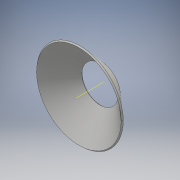
# Autodesk Inventor part: top_roof
Saved by Autodesk Inventor 2016 (Build 200138000, 138)
## iProperties
Created: 2018-04-03
Part Number: top_roof
Material: 一般
Document SubType Name: Sheet Metal
Designer: ASHIJANKEN
Density: 1 g/cm^3
Flat Pattern Width: 18.7953 cm
Flat Pattern Length: 18.7953 cm
Flat Pattern Area: 353.262 cm^2
Sheet Metal Rule: Default_mm
Sheet Metal Width: 187.953 mm
Sheet Metal Length: 187.953 mm
Sheet Metal Area: 35326.162 mm^2
Appearance: 既定
Author: ASHIJANKEN
Autodesk Inventor part; units mm, degrees
ref_plane "YZ Plane" through (0, 0, 0) normal (1, 0, 0) x (0, 1, 0)
ref_plane "XZ Plane" through (0, 0, 0) normal (0, 1, 0) x (-1, 0, 0)
ref_plane "XY Plane" through (0, 0, 0) normal (0, 0, 1) x (1, 0, 0)
sketch "スケッチ1" plane through (0, 0, 0) normal (0, 0, 1) x (1, 0, 0)
  line L0 (0, 0) -> (70, 0)
  line L1 (0, 0) -> (0, 35)
  line L2 (0, 35) -> (30, 35)
  line L3 (30, 35) -> (70, 0)
  line L4 (70, 0) -> (71.6463, 1.8814)
  line L5 (71.6463, 1.8814) -> (31.6463, 36.8814)
  line L6 (31.6463, 36.8814) -> (30, 35)
  dimension "d0" = 70
  dimension "d1" = 35
  dimension "d2" = 30
  dimension "d3" = 2.5
  constraints: 14 end point, 2 horizontal, 2 parallel, 1 perpendicular, 1 vertical
  measures "d0" distance of L0.start L0.end
  measures "d1" distance of L0.start L1.end
  measures "d2" distance of L1.end L2.end
  measures "d3" distance of L4.end L0.end
revolve "回転1" add sketch "スケッチ1" angle 359.9 about axis through (0, 0, 0) along (0, -1, 0) contours L3 L6 L5 L4
equation "\"BendRadius\" = Thickness"
equation "\"BendReliefWidth\" = Thickness"
equation "\"BendReliefDepth\" = 0.5 * Thickness"
equation "\"MinimumRemnant\" = 2 * Thickness"
equation "\"TransitionRadius\" = BendRadius"
equation "\"JacobiRadiusSize\" = BendRadius"
equation "\"GapSize\" = Thickness"
equation "\"Thickness\" = 2.5"
